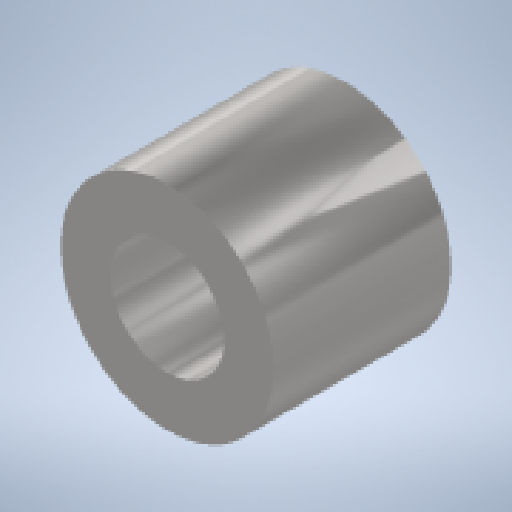
# Autodesk Inventor part: スペーサCU-305
Saved by Autodesk Inventor 2024 (Build 280153000, 153)
## iProperties
Created: 2023-05-27
Part Number: スペーサCU-305
Material: ステンレス鋼
Document SubType Name: Modeling
Designer: yuta2
Density: 8 g/cm^3
Appearance: 半つや出し
Author: yuta2
Autodesk Inventor part; units mm, degrees
ref_plane "YZ Plane" through (0, 0, 0) normal (1, 0, 0) x (0, 1, 0)
ref_plane "XZ Plane" through (0, 0, 0) normal (0, 1, 0) x (-1, 0, 0)
ref_plane "XY Plane" through (0, 0, 0) normal (0, 0, 1) x (1, 0, 0)
sketch "スケッチ1" plane through (0, 0, 0) normal (0, 0, 1) x (1, 0, 0)
  circle A0 centre (0, 0) radius 3
  dimension "d0" = 6
  constraints: 1 centre point, 1 coincident
  measures "d0" diameter of A0
extrude "押し出し1" add sketch "スケッチ1" along normal blind 5
sketch "スケッチ2" plane through (0, 0, 5) normal (0, 0, 1) x (1, 0, 0)
  point P0 (0, 0)
  point P1 (0, 0)
  constraints: 1 coincident
hole "穴1" at (0, 0, 5) direction (0, 0, -1) diameter 3.2 end through all
